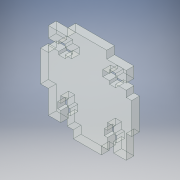
# Autodesk Inventor part: Soporte_Ducto_Rod
Saved by Autodesk Inventor 2019 (Build 230136000, 136)
## iProperties
Created: 2020-04-06
Part Number: Soporte_Ducto_Rod
Material: Generic
Document SubType Name: Modeling
Designer: Jurgen
Density: 1 g/cm^3
Appearance: Clear
Author: Jurgen
Autodesk Inventor part; units mm, degrees
ref_plane "YZ Plane" through (0, 0, 0) normal (1, 0, 0) x (0, 1, 0)
ref_plane "XZ Plane" through (0, 0, 0) normal (0, 1, 0) x (-1, 0, 0)
ref_plane "XY Plane" through (0, 0, 0) normal (0, 0, 1) x (1, 0, 0)
sketch "Sketch1" plane through (0, 0, 0) normal (0, 0, 1) x (1, 0, 0)
  line L0 (-25, -25) -> (25, -25)
  line L1 (25, -25) -> (25, 25)
  line L2 (25, 25) -> (-25, 25)
  line L3 (-25, 25) -> (-25, -25)
  line L4 (-25, -25) -> (25, 25) construction
  line L5 (25, -25) -> (-25, 25) construction
  point P0 (0, 0)
  dimension "d0" = 50
  dimension "d1" = 50
  constraints: 12 end point, 2 midpoint, 2 parallel, 1 horizontal, 1 perpendicular
  measures "d0" distance of L2.end L1.end
  measures "d1" distance of L1.end L0.end
extrude "Extrusion1" add sketch "Sketch1" along normal blind 5
sketch "Sketch2" plane through (0, 0, 5) normal (0, 0, 1) x (1, 0, 0)
  line L0 (-25, -25) -> (25, -25) construction
  line L1 (25, -25) -> (25, 25) construction
  line L2 (25, 25) -> (-25, 25) construction
  line L3 (-25, 25) -> (-25, -25) construction
  line L4 (-25, -25) -> (25, -25) construction
  line L5 (-9, -25) -> (9, -25)
  line L6 (9, -25) -> (9, -30)
  line L7 (9, -30) -> (-9, -30)
  line L8 (-9, -30) -> (-9, -25)
  line L9 (-25, 10) -> (-30, 10)
  line L10 (-30, 10) -> (-30, -10)
  line L11 (-30, -10) -> (-25, -10)
  line L12 (-25, -10) -> (-25, 10)
  line L13 (25, 25) -> (-25, 25) construction
  line L14 (-12.5, 25) -> (12.5, 25)
  line L15 (12.5, 25) -> (12.5, 30)
  line L16 (12.5, 30) -> (-12.5, 30)
  line L17 (-12.5, 30) -> (-12.5, 25)
  line L18 (25, -10) -> (28.5, -10)
  line L19 (28.5, -10) -> (28.5, 10)
  line L20 (28.5, 10) -> (25, 10)
  line L21 (25, 10) -> (25, -10)
  point P0 (0, 0)
  dimension "d4" = 18
  dimension "d5" = 5
  dimension "d6" = 16
  dimension "d7" = 5
  dimension "d8" = 20
  dimension "d9" = 15
  dimension "d10" = 25
  dimension "d11" = 12.5
  dimension "d14" = 3.5
  dimension "d15" = 20
  dimension "d16" = 15
  dimension "d39" = 5
  constraints: 32 end point, 8 parallel, 4 horizontal, 4 perpendicular, 4 point on line
  measures "d4" distance of L6.end L7.end
  measures "d5" distance of L5.end L6.end
  measures "d6" distance between parallel lines of L3 L8
  measures "d7" distance of L11.end L10.end
  measures "d8" distance of L10.end L9.end
  measures "d9" distance between parallel lines of L2 L9
  measures "d10" distance of L16.end L15.end
  measures "d11" distance between parallel lines of L1 L15
  measures "d14" distance of L20.end L19.end
  measures "d15" distance of L19.end L18.end
  measures "d16" distance between parallel lines of L0 L18
  measures "d39" distance of L16.end L14.start
extrude "Extrusion2" add sketch "Sketch2" against normal blind 5
sketch "Sketch3" plane through (0, 0, 5) normal (0, 0, 1) x (1, 0, 0)
  line L0 (-25, -25) -> (-9, -25) construction
  line L1 (-9, -30) -> (-9, -25) construction
  line L2 (9, -30) -> (-9, -30) construction
  line L3 (9, -25) -> (9, -30) construction
  line L4 (9, -25) -> (25, -25) construction
  line L5 (25, -25) -> (25, -10) construction
  line L6 (25, -10) -> (28.5, -10) construction
  line L7 (28.5, -10) -> (28.5, 10) construction
  line L8 (28.5, 10) -> (25, 10) construction
  line L9 (25, 10) -> (25, 25) construction
  line L10 (25, 25) -> (12.5, 25) construction
  line L11 (12.5, 25) -> (12.5, 30) construction
  line L12 (12.5, 30) -> (-12.5, 30) construction
  line L13 (-12.5, 30) -> (-12.5, 25) construction
  line L14 (-12.5, 25) -> (-25, 25) construction
  line L15 (-25, 25) -> (-25, 10) construction
  line L16 (-25, 10) -> (-30, 10) construction
  line L17 (-30, 10) -> (-30, -10) construction
  line L18 (-30, -10) -> (-25, -10) construction
  line L19 (-25, -10) -> (-25, -25) construction
  line L20 (-25, 25) -> (-25, 10) construction
  line L21 (-25, 18) -> (-10, 18) construction
  line L22 (-10, 18) -> (-10, 14) construction
  line L23 (-10, 14) -> (-25, 14) construction
  line L24 (-25, 14) -> (-25, 18) construction
  line L25 (-10, 16) -> (-25, 16) construction
  line L26 (-18.2831, 12) -> (-14.2831, 12) construction
  line L27 (-14.2831, 12) -> (-14.2831, 20) construction
  line L28 (-14.2831, 20) -> (-18.2831, 20) construction
  line L29 (-18.2831, 20) -> (-18.2831, 12) construction
  line L30 (-18.2831, 12) -> (-14.2831, 20) construction
  line L31 (-14.2831, 12) -> (-18.2831, 20) construction
  line L32 (-25, 14) -> (-25, 18)
  line L33 (-25, 18) -> (-18.2831, 18)
  line L34 (-18.2831, 18) -> (-18.2831, 20)
  line L35 (-18.2831, 20) -> (-14.2831, 20)
  line L36 (-14.2831, 20) -> (-14.2831, 18)
  line L37 (-14.2831, 18) -> (-10, 18)
  line L38 (-10, 18) -> (-10, 14)
  line L39 (-10, 14) -> (-14.2831, 14)
  line L40 (-14.2831, 14) -> (-14.2831, 12)
  line L41 (-14.2831, 12) -> (-18.2831, 12)
  line L42 (-18.2831, 12) -> (-18.2831, 14)
  line L43 (-18.2831, 14) -> (-25, 14)
  line L44 (-17, -25) -> (-17, -10) construction
  line L45 (-17, -10) -> (-13, -10) construction
  line L46 (-13, -10) -> (-13, -25) construction
  line L47 (-13, -25) -> (-17, -25) construction
  line L48 (-15, -10) -> (-15, -25) construction
  line L49 (-11, -18.2831) -> (-11, -14.2831) construction
  line L50 (-11, -14.2831) -> (-19, -14.2831) construction
  line L51 (-19, -14.2831) -> (-19, -18.2831) construction
  line L52 (-19, -18.2831) -> (-11, -18.2831) construction
  line L53 (-11, -18.2831) -> (-19, -14.2831) construction
  line L54 (-11, -14.2831) -> (-19, -18.2831) construction
  line L55 (-13, -25) -> (-17, -25)
  line L56 (-17, -25) -> (-17, -18.2831)
  line L57 (-17, -18.2831) -> (-19, -18.2831)
  line L58 (-19, -18.2831) -> (-19, -14.2831)
  line L59 (-19, -14.2831) -> (-17, -14.2831)
  line L60 (-17, -14.2831) -> (-17, -10)
  line L61 (-17, -10) -> (-13, -10)
  line L62 (-13, -10) -> (-13, -14.2831)
  line L63 (-13, -14.2831) -> (-11, -14.2831)
  line L64 (-11, -14.2831) -> (-11, -18.2831)
  line L65 (-11, -18.2831) -> (-13, -18.2831)
  line L66 (-13, -18.2831) -> (-13, -25)
  line L67 (13, -10) -> (17, -10) construction
  line L68 (13, -10) -> (17, -10)
  line L69 (11, -14.2831) -> (13, -14.2831)
  line L70 (13, -14.2831) -> (13, -10)
  line L71 (17, -10) -> (17, -14.2831)
  line L72 (19, -14.2831) -> (11, -14.2831) construction
  line L73 (17, -14.2831) -> (19, -14.2831)
  line L74 (11, -14.2831) -> (11, -18.2831) construction
  line L75 (11, -18.2831) -> (11, -14.2831)
  line L76 (19, -18.2831) -> (11, -14.2831) construction
  line L77 (19, -14.2831) -> (11, -18.2831) construction
  line L78 (19, -18.2831) -> (19, -14.2831) construction
  line L79 (19, -14.2831) -> (19, -18.2831)
  line L80 (13, -25) -> (13, -10) construction
  line L81 (15, -10) -> (15, -25) construction
  line L82 (17, -10) -> (17, -25) construction
  line L83 (13, -18.2831) -> (11, -18.2831)
  line L84 (19, -18.2831) -> (17, -18.2831)
  line L85 (17, -18.2831) -> (17, -25)
  line L86 (17, -25) -> (13, -25) construction
  line L87 (17, -25) -> (13, -25)
  line L88 (13, -25) -> (13, -18.2831)
  line L89 (11, -18.2831) -> (19, -18.2831) construction
  line L90 (25, 14) -> (10, 14) construction
  line L91 (10, 14) -> (10, 18) construction
  line L92 (10, 18) -> (25, 18) construction
  line L93 (25, 18) -> (25, 14) construction
  line L94 (10, 16) -> (25, 16) construction
  line L95 (18.2831, 20) -> (14.2831, 20) construction
  line L96 (14.2831, 20) -> (14.2831, 12) construction
  line L97 (14.2831, 12) -> (18.2831, 12) construction
  line L98 (18.2831, 12) -> (18.2831, 20) construction
  line L99 (18.2831, 20) -> (14.2831, 12) construction
  line L100 (14.2831, 20) -> (18.2831, 12) construction
  line L101 (25, 18) -> (25, 14)
  line L102 (25, 14) -> (18.2831, 14)
  line L103 (18.2831, 14) -> (18.2831, 12)
  line L104 (18.2831, 12) -> (14.2831, 12)
  line L105 (14.2831, 12) -> (14.2831, 14)
  line L106 (14.2831, 14) -> (10, 14)
  line L107 (10, 14) -> (10, 18)
  line L108 (10, 18) -> (14.2831, 18)
  line L109 (14.2831, 18) -> (14.2831, 20)
  line L110 (14.2831, 20) -> (18.2831, 20)
  line L111 (18.2831, 20) -> (18.2831, 18)
  line L112 (18.2831, 18) -> (25, 18)
  point P0 (0, 0)
  point P1 (-16.2831, 16)
  point P2 (-15, -16.2831)
  point P3 (15, -16.2831)
  point P4 (16.2831, 16)
  dimension "d17" = 15
  dimension "d18" = 4
  dimension "d19" = 4
  dimension "d20" = 8
  dimension "d21" = 15
  dimension "d22" = 4
  dimension "d23" = 4
  dimension "d24" = 8
  dimension "d25" = 15
  dimension "d26" = 4
  dimension "d27" = 4
  dimension "d28" = 8
  dimension "d29" = 8
  dimension "d30" = 4
  dimension "d31" = 4
  dimension "d32" = 15
  dimension "d33" = 4
  dimension "d34" = 4
  dimension "d35" = 8
  dimension "d36" = 7
  constraints: 184 end point, 37 point on line, 20 parallel, 16 collinear, 16 midpoint, 16 perpendicular, 2 horizontal, 1 vertical
  measures "d17" distance of L22.end L23.end
  measures "d18" distance of L21.end L22.end
  measures "d19" distance of L28.end L27.end
  measures "d20" distance of L27.end L26.end
  measures "d21" distance of L45.end L46.end
  measures "d22" distance of L45.start L45.end
  measures "d23" distance of L51.end L59.start
  measures "d24" distance of L59.start L50.start
  measures "d25" distance of L82.start L82.end
  measures "d26" distance of L80.end L82.start
  measures "d27" distance of L83.end L74.start
  measures "d28" distance of L74.start L78.end
  measures "d29" distance between parallel lines of L1 L44
  measures "d30" distance between parallel lines of L80 L3
  measures "d31" distance between parallel lines of L16 L23
  measures "d32" distance of L91.end L92.end
  measures "d33" distance of L106.end L91.end
  measures "d34" distance of L97.end L105.start
  measures "d35" distance of L105.start L109.end
  measures "d36" distance between parallel lines of L10 L112
extrude "Extrusion3" cut sketch "Sketch3" against normal blind 5
body "Solid1"
